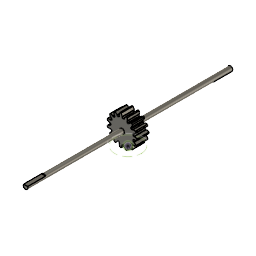
axle (Autodesk Fusion 360 design; units mm, degrees)
part number: 2026-05-16-01-15-47-219
Autodesk Fusion 360 part; units mm, degrees
sketch "Sketch1" plane through (0, 0, 0) normal (0, 0, 1) x (1, 0, 0)
  circle A0 centre (0, 0) radius 12.5 construction
  dimension "d1" = 25
  constraint coincident A0.centre origin
  measures "d1" diameter of A0
sketch "Base Circle" plane through (0, 0, 0) normal (0, 0, 1) x (1, 0, 0)
  circle A0 centre (0, 0) radius 9.3279
  circle A1 centre (0, 0) radius 1.15
extrude "Extrude1" add sketch "Base Circle" along normal blind 10
sketch "Gear Tooth" plane through (0, 0, 0) normal (0, 0, 1) x (1, 0, 0)
  spline S0 degree 5 poles (10.2902, -1.2369) (10.2964, -1.2376) (10.3089, -1.2389) (10.3277, -1.2404) (10.3528, -1.2412) (10.3842, -1.2409) (10.4157, -1.2395) (10.4473, -1.2374) (10.4789, -1.2351) (10.5106, -1.2325) (10.5422, -1.2296) (10.5739, -1.2264) (10.6056, -1.2228) (10.6373, -1.2187) (10.6691, -1.2141) (10.7008, -1.209) (10.7326, -1.2035) (10.7644, -1.1976) (10.7962, -1.1915) (10.828, -1.1851) (10.8597, -1.1784) (10.8915, -1.1714) (10.9233, -1.1641) (10.9551, -1.1564) (10.9869, -1.1485) (11.0187, -1.1402) (11.0505, -1.1317) (11.0823, -1.1229) (11.114, -1.1138) (11.1458, -1.1044) (11.1776, -1.0948) (11.2093, -1.085) (11.241, -1.0748) (11.2727, -1.0645) (11.3045, -1.0538) (11.3361, -1.0429) (11.3678, -1.0318) (11.3995, -1.0204) (11.4311, -1.0087) (11.4627, -0.9969) (11.4943, -0.9847) (11.5259, -0.9724) (11.5575, -0.9598) (11.589, -0.947) (11.6206, -0.934) (11.6521, -0.9207) (11.6835, -0.9072) (11.715, -0.8935) (11.7464, -0.8796) (11.7778, -0.8654) (11.8091, -0.8511) (11.8405, -0.8365) (11.8718, -0.8217) (11.9031, -0.8067) (11.9343, -0.7914) (11.9655, -0.776) (11.9967, -0.7603) (12.0279, -0.7445) (12.059, -0.7284) (12.0901, -0.7122) (12.1211, -0.6957) (12.1521, -0.679) (12.1831, -0.6622) (12.214, -0.6451) (12.2449, -0.6278) (12.2758, -0.6103) (12.3066, -0.5927) (12.3374, -0.5748) (12.3682, -0.5567) (12.3988, -0.5385) (12.4295, -0.52) (12.454, -0.5051) (12.4723, -0.4939) (12.4846, -0.4863) (12.4907, -0.4825) knots 0 0 0 0 0 0 0.01428571 0.02857143 0.04285714 0.05714286 0.07142857 0.08571429 0.1 0.11428571 0.12857143 0.14285714 0.15714286 0.17142857 0.18571429 0.2 0.21428571 0.22857143 0.24285714 0.25714286 0.27142857 0.28571429 0.3 0.31428571 0.32857143 0.34285714 0.35714286 0.37142857 0.38571429 0.4 0.41428571 0.42857143 0.44285714 0.45714286 0.47142857 0.48571429 0.5 0.51428571 0.52857143 0.54285714 0.55714286 0.57142857 0.58571429 0.6 0.61428571 0.62857143 0.64285714 0.65714286 0.67142857 0.68571429 0.7 0.71428571 0.72857143 0.74285714 0.75714286 0.77142857 0.78571429 0.8 0.81428571 0.82857143 0.84285714 0.85714286 0.87142857 0.88571429 0.9 0.91428571 0.92857143 0.94285714 0.95714286 0.97142857 0.98571429 1 1 1 1 1 1
  spline S1 degree 5 poles (10.2902, 1.2369) (10.2964, 1.2376) (10.3089, 1.2389) (10.3277, 1.2404) (10.3528, 1.2412) (10.3842, 1.2409) (10.4157, 1.2395) (10.4473, 1.2374) (10.4789, 1.2351) (10.5106, 1.2325) (10.5422, 1.2296) (10.5739, 1.2264) (10.6056, 1.2228) (10.6373, 1.2187) (10.6691, 1.2141) (10.7008, 1.209) (10.7326, 1.2035) (10.7644, 1.1976) (10.7962, 1.1915) (10.828, 1.1851) (10.8597, 1.1784) (10.8915, 1.1714) (10.9233, 1.1641) (10.9551, 1.1564) (10.9869, 1.1485) (11.0187, 1.1402) (11.0505, 1.1317) (11.0823, 1.1229) (11.114, 1.1138) (11.1458, 1.1044) (11.1776, 1.0948) (11.2093, 1.085) (11.241, 1.0748) (11.2727, 1.0645) (11.3045, 1.0538) (11.3361, 1.0429) (11.3678, 1.0318) (11.3995, 1.0204) (11.4311, 1.0087) (11.4627, 0.9969) (11.4943, 0.9847) (11.5259, 0.9724) (11.5575, 0.9598) (11.589, 0.947) (11.6206, 0.934) (11.6521, 0.9207) (11.6835, 0.9072) (11.715, 0.8935) (11.7464, 0.8796) (11.7778, 0.8654) (11.8091, 0.8511) (11.8405, 0.8365) (11.8718, 0.8217) (11.9031, 0.8067) (11.9343, 0.7914) (11.9655, 0.776) (11.9967, 0.7603) (12.0279, 0.7445) (12.059, 0.7284) (12.0901, 0.7122) (12.1211, 0.6957) (12.1521, 0.679) (12.1831, 0.6622) (12.214, 0.6451) (12.2449, 0.6278) (12.2758, 0.6103) (12.3066, 0.5927) (12.3374, 0.5748) (12.3682, 0.5567) (12.3988, 0.5385) (12.4295, 0.52) (12.454, 0.5051) (12.4723, 0.4939) (12.4846, 0.4863) (12.4907, 0.4825) knots 0 0 0 0 0 0 0.01428571 0.02857143 0.04285714 0.05714286 0.07142857 0.08571429 0.1 0.11428571 0.12857143 0.14285714 0.15714286 0.17142857 0.18571429 0.2 0.21428571 0.22857143 0.24285714 0.25714286 0.27142857 0.28571429 0.3 0.31428571 0.32857143 0.34285714 0.35714286 0.37142857 0.38571429 0.4 0.41428571 0.42857143 0.44285714 0.45714286 0.47142857 0.48571429 0.5 0.51428571 0.52857143 0.54285714 0.55714286 0.57142857 0.58571429 0.6 0.61428571 0.62857143 0.64285714 0.65714286 0.67142857 0.68571429 0.7 0.71428571 0.72857143 0.74285714 0.75714286 0.77142857 0.78571429 0.8 0.81428571 0.82857143 0.84285714 0.85714286 0.87142857 0.88571429 0.9 0.91428571 0.92857143 0.94285714 0.95714286 0.97142857 0.98571429 1 1 1 1 1 1
  arc A0 (12.4907, -0.4825) -> (12.4907, 0.4825) centre (0, 0) ccw
  line L0 (9.2514, -1.112) -> (10.2902, -1.2369)
  line L1 (9.2514, 1.112) -> (10.2902, 1.2369)
  line L2 (9.2514, -1.112) -> (9.2514, 1.112)
  point P0 (10.4437, -1.2376)
  point P1 (10.599, -1.2235)
  point P2 (10.7553, -1.1992)
  point P3 (10.9123, -1.1666)
  point P4 (11.0699, -1.1263)
  point P5 (11.2278, -1.079)
  point P6 (11.3861, -1.0252)
  point P7 (11.5444, -0.965)
  point P8 (11.7028, -0.8988)
  point P9 (11.861, -0.8267)
  point P10 (12.019, -0.749)
  point P11 (12.1767, -0.6656)
  point P12 (12.334, -0.5768)
  point P13 (10.4437, 1.2376)
  point P14 (10.599, 1.2235)
  point P15 (10.7553, 1.1992)
  point P16 (10.9123, 1.1666)
  point P17 (11.0699, 1.1263)
  point P18 (11.2278, 1.079)
  point P19 (11.3861, 1.0252)
  point P20 (11.5444, 0.965)
  point P21 (11.7028, 0.8988)
  point P22 (11.861, 0.8267)
  point P23 (12.019, 0.749)
  point P24 (12.1767, 0.6656)
  point P25 (12.334, 0.5768)
extrude "Extrude2" add sketch "Gear Tooth" along normal blind 10
fillet "Fillet1" radius 0.8 2 edges at (9.2613, -1.1132, 5) (9.2613, 1.1132, 5)
pattern_circular "C-Pattern1" count 15 over 360 about axis through (0, 0, 0) along (0, 0, 1) of "Extrude2", "Fillet1"
sketch "Diametrial Pitch Circle" plane through (0, 0, 0) normal (0, 0, 1) x (1, 0, 0)
  circle A0 centre (0, 0) radius 11.0294 construction
sketch "Sketch5" plane through (0, 0, 0) normal (0, 0, 1) x (1, 0, 0)
  circle A0 centre (0, 0) radius 1.15
  dimension "d10" = 2.3
  constraint coincident A0.centre origin
  measures "d10" diameter of A0
extrude "Extrude3" add sketch "Sketch5" along normal blind 10
sketch "Sketch6" plane through (0, 0, 0) normal (0, 0, 1) x (1, 0, 0)
  circle A0 centre (0, 0) radius 2
  line L0 (1.7319, -1.0003) -> (-1.7676, -0.9358)
  dimension "d13" = 4
  dimension "d14" = 3.5
  constraint coincident A0.centre origin
  constraint coincident A0 L0.start
  constraint coincident A0 L0.end
  measures "d13" diameter of A0
  measures "d14" distance of L0.start L0.end
move_body "Move1" bodies 1 to x (1, 0, 0) y (0, 1, 0) z (0, 0, 1) at (0, 0, 80)
extrude "Extrude4" add sketch "Sketch6" along normal blind 80
extrude "Extrude5" cut sketch "Sketch6" along normal blind 15 contours A0 L0 picked at (-0.551, -1.0376)
move_body "Move2" bodies 1 to x (1, 0, 0) y (0, -1, 0) z (0, 0, -1) at (0, 0.0546, 170)
extrude "Extrude6" add sketch "Sketch6" along normal blind 80
extrude "Extrude7" cut sketch "Sketch6" along normal blind 15 contours A0 L0 picked at (-0.551, -1.0376)
move_body "Move3" bodies 1 to x (1, 0, 0) y (0, 0, 1) z (0, -1, 0) at (0, 0, 0)
move_body "Move4" bodies 1 to x (1, 0, 0) y (0, 1, 0) z (0, 0, 1) at (0, 85, 0)
move_body "Move5" bodies 1 to x (1, 0, 0) y (0, 1, 0) z (0, 0, 1) at (0, 0, 13)
named bodies: "Spur Gear (15 teeth)"
